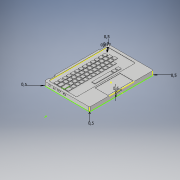
# Autodesk Inventor part: UnderdelDatorchassi
Saved by Autodesk Inventor 2018 (Build 220112000, 112)
## iProperties
Created: 2017-11-21
Part Number: UnderdelDatorchassi
Material: Generic
Document SubType Name: Modeling
Designer: 17riwi
Density: 1 g/cm^3
Appearance: Default
Author: 17riwi
## iProperties of the stored document UnderdelDatorchassi_3DPrint.ipt
Created: 2017-12-14
Part Number: UnderdelDatorchassi_3DPrint
Material: Generic
Document SubType Name: Modeling
Designer: 17riwi
Density: 1 g/cm^3
Appearance: Default
Author: 17riwi
Autodesk Inventor part; units mm, degrees
(part 1 of 2)
ref_plane "YZ Plane" through (0, 0, 0) normal (1, 0, 0) x (0, 1, 0)
ref_plane "XZ Plane" through (0, 0, 0) normal (0, 1, 0) x (-1, 0, 0)
ref_plane "XY Plane" through (0, 0, 0) normal (0, 0, 1) x (1, 0, 0)
sketch "Sketch1" plane through (0, 0, 0) normal (0, 1, 0) x (-1, 0, 0)
  point P0 (0, 0)
sketch "Sketch2" plane through (0, 0, 0) normal (0, 1, 0) x (-1, 0, 0)
  line L0 (-50.8, 147.4) -> (-50.8, -147.4)
  line L1 (-45.8, -152.4) -> (160.1, -152.4)
  line L2 (160.1, 152.4) -> (-45.8, 152.4)
  arc A0 (-45.8, 152.4) -> (-50.8, 147.4) centre (-45.8, 147.4) ccw
  arc A1 (-50.8, -147.4) -> (-45.8, -152.4) centre (-45.8, -147.4) ccw
  arc A2 (160.1, -152.4) -> (165.1, -147.4) centre (160.1, -147.4) ccw
  arc A3 (165.1, 147.4) -> (160.1, 152.4) centre (160.1, 147.4) ccw
  line L3 (160.0443, 130.175) -> (165.1, 130.175)
  line L4 (165.1, 130.175) -> (168.275, 130.175)
  line L5 (168.2193, 130.0929) -> (168.2193, 104.6929)
  line L6 (168.2193, 104.6929) -> (165.1, 104.6929)
  line L7 (160.0443, 104.6929) -> (160.0443, 130.175)
  line L8 (165.1, 130.175) -> (165.1, 147.4)
  line L9 (165.1, 104.6929) -> (160.0443, 104.6929)
  line L10 (161.6875, -106.4446) -> (166.6318, -106.4446)
  line L11 (166.6318, -106.4446) -> (169.8625, -106.4446)
  line L12 (169.8625, -106.4446) -> (169.8625, -131.7625)
  line L13 (169.8625, -131.7625) -> (166.6875, -131.7625)
  line L14 (161.6875, -131.7625) -> (161.6875, -106.4446)
  line L15 (166.6875, -131.7625) -> (161.6875, -131.7625)
  line L16 (171.45, -131.6395) -> (171.45, -131.7625)
  line L17 (165.1, -147.4) -> (165.1, -131.7625)
  line L18 (165.1, -106.4446) -> (165.1, 104.6929)
  line L19 (22.225, -126.9496) -> (22.225, -131.7625)
  line L20 (22.1693, -44.5321) -> (22.1693, -106.4446)
  line L21 (22.225, -131.7625) -> (22.225, -126.9496)
  line L22 (22.1693, -106.4446) -> (22.1693, 104.6929)
  line L23 (22.225, 130.175) -> (22.225, 134.2875)
  line L24 (153.8637, 11.0475) -> (153.8637, 132.4231)
  line L25 (146.8637, 141.2875) -> (29.225, 141.2875)
  line L26 (22.225, 134.2875) -> (22.225, -126.9496)
  arc A4 (153.7963, -127.9188) -> (153.8637, -126.9496) centre (146.8637, -126.9496) ccw
  arc A5 (29.225, 141.2875) -> (22.225, 134.2875) centre (29.225, 134.2875) ccw
  line L27 (-45.8, -60.325) -> (15.875, -60.325)
  line L28 (-19.5021, 60.09) -> (15.875, 60.09)
  line L29 (15.875, 60.09) -> (15.875, -60.325)
  line L30 (-19.05, -60.325) -> (-45.8, -60.325)
  line L31 (-45.8, -60.325) -> (-45.8, 60.09)
  line L32 (-45.8, 60.09) -> (15.875, 60.09)
  line L33 (-14.9625, 60.325) -> (15.875, 60.325)
  line L34 (-9.525, -60.325) -> (15.875, -60.325)
  line L35 (15.875, -60.325) -> (15.875, 60.325)
  line L36 (22.225, -132.5813) -> (22.225, -131.7625)
  line L37 (22.225, -44.45) -> (22.225, -106.3625)
  line L38 (22.225, -131.7625) -> (22.225, -132.5813)
  line L39 (22.225, -106.3625) -> (22.225, 104.775)
  line L40 (22.225, 130.175) -> (22.225, 134.2875)
  line L41 (148.575, -139.5812) -> (29.225, -139.5812)
  line L42 (155.575, -132.5813) -> (155.575, 134.2875)
  line L43 (148.575, 141.2875) -> (29.225, 141.2875)
  line L44 (22.225, 134.2875) -> (22.225, -132.5813)
  arc A6 (148.575, -139.5812) -> (155.575, -132.5813) centre (148.575, -132.5813) ccw
  arc A7 (22.225, -132.5813) -> (29.225, -139.5812) centre (29.225, -132.5813) ccw
  arc A8 (29.225, 141.2875) -> (22.225, 134.2875) centre (29.225, 134.2875) ccw
  arc A9 (155.575, 134.2875) -> (148.575, 141.2875) centre (148.575, 134.2875) ccw
  line L45 (26.9875, 60.325) -> (26.9875, 60.09)
  line L46 (147.2195, 137.8825) -> (31.8081, 137.8825)
  arc A10 (146.8637, -135.8473) -> (153.7963, -127.9188) centre (147.127, -129.0825) ccw
  arc A11 (31.8081, 137.8825) -> (25.0381, 131.1125) centre (31.8081, 131.1125) ccw
  line L47 (26.9875, 60.325) -> (26.9875, 60.09)
  line L48 (146.8637, -135.8473) -> (33.9358, -135.8473)
  arc A12 (25.0381, -126.9496) -> (33.9358, -135.8473) centre (33.9358, -126.9496) ccw
  arc A13 (33.9875, 282.575) -> (31.3881, 282.0745) centre (33.9875, 275.575) ccw
  line L49 (25.0381, 131.1125) -> (25.0381, -126.9496)
  arc A14 (153.8637, 132.4231) -> (147.2195, 137.8825) centre (147.0348, 130.8849) ccw
  line L50 (153.8637, -126.9449) -> (153.8637, 1.7361)
  line L51 (153.9875, 60.09) -> (153.9875, 60.325)
  line L52 (153.8637, 1.7361) -> (153.8637, 11.0475)
  point P0 (0, 0)
  point P1 (22.225, -133.9496)
  point P2 (153.8637, 134.2875)
  point P3 (22.225, -139.5812)
  point P4 (26.9875, 1.7063)
  point P5 (26.9875, 1.7063)
  dimension "d0" = 5
  dimension "d1" = 5
  dimension "d2" = 5
  dimension "d3" = 5
  dimension "d5" = 7
  dimension "d6" = 6.77
  constraints: 106 end point, 31 point on circle, 26 tangent, 23 perpendicular, 19 point on line, 15 centre point, 6 equal radius, 6 vertical, 4 horizontal, 4 parallel, 2 collinear, 1 coincident
  measures "d0" radius of A0
  measures "d1" radius of A1
  measures "d2" radius of A2
  measures "d3" radius of A3
  measures "d5" radius of A6
  measures "d6" radius of A10
extrude "Extrusion1" add sketch "Sketch2" along normal blind 1 contours L31 L32 L28 L29 L27
extrude "Extrusion2" cut sketch "Sketch2" along normal blind 18 contours L31 L32 L28 L29 L27
extrude "Extrusion3" add sketch "Sketch2" along normal blind 19 contours A0 L2 A3 L8 L3 L7 L9 L18 L10 L14 L15 L17 A2 L1 A1 L0
extrude "Extrusion4" add sketch "Sketch2" along normal blind 18 contours L26 L23 A5 L25 L43 A9 L42 A6 L41 A7 L36 L19
extrude "Extrusion5" cut sketch "Sketch2" against normal blind 1 contours L26 L23 A5 L25 L43 A9 L42 A6 L41 A7 L36 L19
extrude "Extrusion6" add sketch "Sketch2" along normal blind 18 contours L31 L32 L28 L29 L27
extrude "Extrusion7" cut sketch "Sketch2" against normal blind 19 contours L26 L23 A5 L25 L43 A9 L42 A6 L41 A7 L36 L19
extrude "Extrusion8" cut sketch "Sketch2" along normal blind 1.5375 contours L26 L23 A5 L25 L43 A9 L42 A6 L41 A7 L36 L19
extrude "Extrusion9" add sketch "Sketch2" against normal blind 1.5375 contours L26 L23 A5 L25 L43 A9 L42 A6 L41 A7 L36 L19
boundary_patch "Boundary Patch1"
boundary_patch "Boundary Patch2"
sketch "Sketch3" plane through (-160.1, 0, 152.4) normal (0, 0, 1) x (1, 0, 0)
  circle A0 centre (19.8438, 12.7) radius 3.9888
  line L0 (36.5125, 12.7) -> (36.5125, 8.7112)
  line L1 (36.5125, 8.7112) -> (46.0375, 8.7112)
  line L2 (46.0375, 8.7112) -> (46.0375, 12.7)
  line L3 (46.0375, 12.7) -> (36.5125, 12.7)
  line L4 (58.7375, 8.7112) -> (55.5625, 12.7)
  line L5 (55.5625, 12.7) -> (55.5625, 14.6944)
  line L6 (58.7375, 8.7112) -> (68.2625, 8.7112)
  line L7 (68.2625, 8.7112) -> (71.4375, 12.7)
  line L8 (71.4375, 12.7) -> (71.4375, 14.6944)
  line L9 (71.4375, 14.6944) -> (55.5625, 14.6944)
  line L10 (84.1375, 14.6944) -> (84.1375, 8.7112)
  line L11 (84.1375, 8.7112) -> (96.8375, 8.7112)
  line L12 (96.8375, 8.7112) -> (96.8375, 14.6944)
  line L13 (96.8375, 14.6944) -> (84.1375, 14.6944)
  point P0 (160.1, 0)
  constraints: 28 end point, 7 perpendicular, 1 centre point, 1 horizontal, 1 vertical
extrude "Extrusion10" cut sketch "Sketch3" against normal blind 5
sketch3d "3D Sketch2"
sketch "Sketch4" plane through (45.8, 0, -152.4) normal (0, 0, -1) x (-1, 0, 0)
  line L0 (0, 19) -> (205.9, 19) projected
  line L1 (192.1104, 15.875) -> (192.1104, 9.525)
  line L2 (192.1104, 9.525) -> (183.6418, 9.525)
  circle A0 centre (186.0563, 12.7) radius 3.9888 projected
  line L3 (183.6418, 15.875) -> (192.1104, 15.875)
  line L4 (183.6418, 15.875) -> (183.6418, 9.525)
  point P0 (45.8, 0)
  constraints: 8 end point, 2 point on circle, 1 parallel, 1 perpendicular, 1 vertical
extrude "Extrusion11" cut sketch "Sketch4" against normal blind 5 contours L1 L2 A0 L3 | A0 L2 L4 L3
sketch "Sketch5" plane through (45.8, 0, -152.4) normal (0, 0, -1) x (-1, 0, 0)
  point P0 (45.8, 0)
sketch "Sketch6" plane through (0, 19, 0) normal (0, 1, 0) x (1, 0, 0)
  point P0 (0, 0)
sketch "Sketch7" plane through (50.8, 0, 147.4) normal (1, 0, 0) x (0, 0, -1)
  line L0 (87.31, 19) -> (207.725, 19) projected
  line L1 (147.5175, 19) -> (147.5175, 13)
  line L2 (294.8, 0) -> (294.8, 19) projected
  line L3 (-5, 0) -> (-5, 19) projected
  point P0 (147.4, 0)
  dimension "d36" = 6
  constraints: 2 end point, 1 midpoint, 1 vertical
  measures "d36" distance of L1.start L1.end
sketch "Sketch8" plane through (0, 18, 0) normal (0, 1, 0) x (1, 0, 0)
  line L0 (-155.575, 132.5813) -> (-155.575, -134.2875) projected
  point P0 (0, 0)
sketch "Sketch9" plane through (0, 18, 0) normal (0, 1, 0) x (1, 0, 0)
  point P0 (0, 0)
sketch "Sketch10" plane through (0, 18, 0) normal (0, 1, 0) x (1, 0, 0)
  point P0 (0, 0)
sketch "Sketch11" plane through (0, 18, 0) normal (0, 1, 0) x (1, 0, 0)
  point P0 (0, 0)
sketch "Sketch12" plane through (0, 18, 0) normal (0, 1, 0) x (1, 0, 0)
  point P0 (0, 0)
sketch "Sketch13" plane through (0, 18, 0) normal (0, 1, 0) x (1, 0, 0)
  line L0 (-136.525, 106.3625) -> (-120.65, 106.3625)
  line L1 (-120.65, 106.3625) -> (-120.65, 90.4875)
  line L2 (-120.65, 90.4875) -> (-136.525, 90.4875)
  line L3 (-136.525, 90.4875) -> (-136.525, 106.3625)
  line L4 (-136.525, 88.9) -> (-120.65, 88.9)
  line L5 (-120.65, 88.9) -> (-120.65, 73.025)
  line L6 (-120.65, 73.025) -> (-136.525, 73.025)
  line L7 (-136.525, 73.025) -> (-136.525, 88.9)
  line L8 (-136.525, 69.85) -> (-120.65, 69.85)
  line L9 (-120.65, 69.85) -> (-120.65, 53.975)
  line L10 (-120.65, 53.975) -> (-136.525, 53.975)
  line L11 (-136.525, 53.975) -> (-136.525, 69.85)
  line L12 (-136.525, 50.8) -> (-120.65, 50.8)
  line L13 (-120.65, 50.8) -> (-120.65, 34.925)
  line L14 (-120.65, 34.925) -> (-136.525, 34.925)
  line L15 (-136.525, 34.925) -> (-136.525, 50.8)
  line L16 (-136.525, 33.3375) -> (-120.65, 33.3375)
  line L17 (-120.65, 33.3375) -> (-120.65, 17.4625)
  line L18 (-120.65, 17.4625) -> (-136.525, 17.4625)
  line L19 (-136.525, 17.4625) -> (-136.525, 33.3375)
  line L20 (-136.525, 15.875) -> (-120.65, 15.875)
  line L21 (-120.65, 15.875) -> (-120.65, 0)
  line L22 (-120.65, 0) -> (-136.525, 0)
  line L23 (-136.525, 0) -> (-136.525, 15.875)
  line L24 (-136.525, -1.5875) -> (-120.65, -1.5875)
  line L25 (-120.65, -1.5875) -> (-120.65, -17.4625)
  line L26 (-120.65, -17.4625) -> (-136.525, -17.4625)
  line L27 (-136.525, -17.4625) -> (-136.525, -1.5875)
  line L28 (-136.525, -19.05) -> (-120.65, -19.05)
  line L29 (-120.65, -19.05) -> (-120.65, -34.925)
  line L30 (-120.65, -34.925) -> (-136.525, -34.925)
  line L31 (-136.525, -34.925) -> (-136.525, -19.05)
  line L32 (-136.525, -38.1) -> (-120.65, -38.1)
  line L33 (-120.65, -38.1) -> (-120.65, -53.975)
  line L34 (-120.65, -53.975) -> (-136.525, -53.975)
  line L35 (-136.525, -53.975) -> (-136.525, -38.1)
  line L36 (-136.525, -55.5625) -> (-120.65, -55.5625)
  line L37 (-120.65, -55.5625) -> (-120.65, -71.4375)
  line L38 (-120.65, -71.4375) -> (-136.525, -71.4375)
  line L39 (-136.525, -71.4375) -> (-136.525, -55.5625)
  line L40 (-136.525, -74.6125) -> (-120.65, -74.6125)
  line L41 (-120.65, -74.6125) -> (-120.65, -90.4875)
  line L42 (-120.65, -90.4875) -> (-136.525, -90.4875)
  line L43 (-136.525, -90.4875) -> (-136.525, -74.6125)
  line L44 (-136.525, -92.075) -> (-120.65, -92.075)
  line L45 (-120.65, -92.075) -> (-120.65, -107.95)
  line L46 (-120.65, -107.95) -> (-136.525, -107.95)
  line L47 (-136.525, -107.95) -> (-136.525, -92.075)
  line L48 (-136.525, -109.5375) -> (-120.65, -109.5375)
  line L49 (-120.65, -109.5375) -> (-120.65, -125.4125)
  line L50 (-120.65, -125.4125) -> (-136.525, -125.4125)
  line L51 (-136.525, -125.4125) -> (-136.525, -109.5375)
  point P0 (0, 0)
  constraints: 104 end point, 26 parallel, 18 point on line, 13 horizontal, 13 perpendicular
extrude "Extrusion12" cut sketch "Sketch13" against normal blind 5
sketch "Sketch14" plane through (0, 18, 0) normal (0, 1, 0) x (1, 0, 0)
  line L0 (-120.65, 50.8) -> (-120.65, 34.925) projected
  line L1 (-117.475, 39.6875) -> (-117.475, 20.6875)
  line L2 (-117.475, 15.6875) -> (-117.475, 1.6875)
  line L3 (-117.475, -3.3125) -> (-117.475, -17.3125)
  line L4 (-117.475, -22.3125) -> (-117.475, -36.3125)
  line L5 (-117.475, -41.3125) -> (-117.475, -55.3125)
  line L6 (-117.475, -60.3125) -> (-117.475, -74.3125)
  line L7 (-117.475, -79.3125) -> (-117.475, -93.223)
  line L8 (-117.475, -93.3125) -> (-117.475, -88.3125)
  line L9 (-117.475, -102.3125) -> (-117.475, -112.223)
  line L10 (-102.475, -102.3125) -> (-102.475, -97.3125)
  line L11 (-102.475, 111.125) -> (-117.475, 111.125)
  line L12 (-117.475, 111.125) -> (-102.475, 111.125)
  line L13 (-117.475, 96.8375) -> (-102.475, 96.8375)
  line L14 (-117.475, 92.075) -> (-102.475, 92.075)
  line L15 (-117.475, 77.7875) -> (-102.475, 77.7875)
  line L16 (-117.475, 73.025) -> (-102.475, 73.025)
  line L17 (-117.475, 58.7375) -> (-102.475, 58.7375)
  line L18 (-117.475, 39.6875) -> (-102.475, 39.6875)
  line L19 (-117.475, 34.6875) -> (-102.475, 34.6875)
  line L20 (-117.475, 20.6875) -> (-102.475, 20.6875)
  line L21 (-117.475, 15.6875) -> (-102.475, 15.6875)
  line L22 (-117.475, 1.6875) -> (-102.475, 1.6875)
  line L23 (-117.475, -3.3125) -> (-102.475, -3.3125)
  line L24 (-117.475, -17.3125) -> (-102.475, -17.3125)
  line L25 (-117.475, -22.3125) -> (-102.475, -22.3125)
  line L26 (-117.475, -36.3125) -> (-102.475, -36.3125)
  line L27 (-117.475, -41.3125) -> (-102.475, -41.3125)
  line L28 (-117.475, -55.3125) -> (-102.475, -55.3125)
  line L29 (-117.475, -60.3125) -> (-102.475, -60.3125)
  line L30 (-117.475, -74.3125) -> (-102.475, -74.3125)
  line L31 (-117.475, -79.3125) -> (-102.475, -79.3125)
  line L32 (-98.475, 110.777) -> (-98.475, 101.777)
  line L33 (-98.475, -107.223) -> (-83.475, -107.223)
  line L34 (-98.475, -107.223) -> (-98.475, -93.3125)
  line L35 (-98.475, -88.223) -> (-98.475, -74.3125)
  line L36 (-98.475, -69.223) -> (-98.475, -55.223)
  line L37 (-98.475, -50.223) -> (-98.475, -36.223)
  line L38 (-98.475, -31.223) -> (-98.475, -17.3125)
  line L39 (-98.475, -12.223) -> (-98.475, 1.777)
  line L40 (-98.475, 6.777) -> (-98.475, 20.777)
  line L41 (-98.475, 25.777) -> (-98.475, 39.777)
  line L42 (-98.475, 44.777) -> (-98.475, 58.777)
  line L43 (-98.475, 63.777) -> (-98.475, 77.777)
  line L44 (-98.475, 77.777) -> (-98.475, 77.7875)
  line L45 (-98.475, 82.777) -> (-98.475, 96.777)
  line L46 (-98.475, 97.777) -> (-98.475, 82.777)
  line L47 (-98.475, 82.777) -> (-98.475, 96.777)
  line L48 (-98.475, 101.777) -> (-98.475, 115.777)
  line L49 (-98.475, 115.777) -> (-83.475, 115.777)
  line L50 (-98.475, 101.777) -> (-83.475, 101.777)
  line L51 (-83.475, 96.777) -> (-98.475, 96.777)
  line L52 (-98.475, 82.777) -> (-83.475, 82.777)
  line L53 (-83.475, 77.777) -> (-98.475, 77.777)
  line L54 (-98.475, 63.777) -> (-83.475, 63.777)
  line L55 (-83.475, 58.777) -> (-98.475, 58.777)
  line L56 (-98.475, 44.777) -> (-83.475, 44.777)
  line L57 (-83.475, 39.777) -> (-98.475, 39.777)
  line L58 (-98.475, 25.777) -> (-83.475, 25.777)
  line L59 (-83.475, 20.777) -> (-98.475, 20.777)
  line L60 (-98.475, 6.777) -> (-83.475, 6.777)
  line L61 (-83.475, 1.777) -> (-98.475, 1.777)
  line L62 (-98.475, -12.223) -> (-83.475, -12.223)
  line L63 (-83.475, -17.223) -> (-98.475, -17.223)
  line L64 (-98.475, -31.223) -> (-83.475, -31.223)
  line L65 (-83.475, -36.223) -> (-98.475, -36.223)
  line L66 (-98.475, -50.223) -> (-83.475, -50.223)
  line L67 (-83.475, -55.223) -> (-98.475, -55.223)
  line L68 (-98.475, -69.223) -> (-83.475, -69.223)
  line L69 (-98.475, -88.223) -> (-83.475, -88.223)
  line L70 (-83.475, -93.223) -> (-98.475, -93.223)
  line L71 (-98.475, -112.223) -> (-83.475, -112.223)
  line L72 (-83.475, -112.223) -> (-83.475, -138.223)
  line L73 (-83.475, -138.223) -> (-98.475, -138.223)
  line L74 (-98.475, -138.223) -> (-98.475, -112.223)
  line L75 (-90.975, 119.936) -> (-83.475, 119.936)
  line L76 (-92.075, 119.936) -> (-83.475, 119.936)
  line L77 (-83.475, 119.936) -> (-83.475, 132.936)
  line L78 (-83.475, 132.936) -> (-117.475, 132.936)
  line L79 (-117.475, 132.936) -> (-117.475, 115.936)
  line L80 (-117.475, 115.936) -> (-117.475, 132.936)
  line L81 (-83.475, -107.223) -> (-98.475, -107.223)
  line L82 (-98.475, -107.223) -> (-98.475, -93.223)
  line L83 (-98.475, -93.223) -> (-83.475, -93.223)
  line L84 (-83.475, -93.223) -> (-83.475, -107.223)
  line L85 (-83.475, -88.223) -> (-98.475, -88.223)
  line L86 (-98.475, -88.223) -> (-98.475, -74.223)
  line L87 (-98.475, -74.223) -> (-83.475, -74.223)
  line L88 (-83.475, -74.223) -> (-83.475, -88.223)
  line L89 (-83.475, -69.223) -> (-98.475, -69.223)
  line L90 (-98.475, -69.223) -> (-98.475, -55.223)
  line L91 (-98.475, -55.223) -> (-83.475, -55.223)
  line L92 (-83.475, -55.223) -> (-83.475, -69.223)
  line L93 (-83.475, -50.223) -> (-98.475, -50.223)
  line L94 (-98.475, -50.223) -> (-98.475, -36.223)
  line L95 (-98.475, -36.223) -> (-83.475, -36.223)
  line L96 (-83.475, -36.223) -> (-83.475, -50.223)
  line L97 (-83.475, -31.223) -> (-98.475, -31.223)
  line L98 (-98.475, -31.223) -> (-98.475, -17.223)
  line L99 (-98.475, -17.223) -> (-83.475, -17.223)
  line L100 (-83.475, -17.223) -> (-83.475, -31.223)
  line L101 (-83.475, -12.223) -> (-98.475, -12.223)
  line L102 (-98.475, -12.223) -> (-98.475, 1.777)
  line L103 (-98.475, 1.777) -> (-83.475, 1.777)
  line L104 (-83.475, 1.777) -> (-83.475, -12.223)
  line L105 (-83.475, 6.777) -> (-98.475, 6.777)
  line L106 (-98.475, 6.777) -> (-98.475, 20.6875)
  line L107 (-98.475, 20.777) -> (-83.475, 20.777)
  line L108 (-83.475, 20.777) -> (-83.475, 20.6875)
  line L109 (-83.475, 25.777) -> (-98.475, 25.777)
  line L110 (-98.475, 25.777) -> (-98.475, 39.777)
  line L111 (-98.475, 39.777) -> (-83.475, 39.777)
  line L112 (-83.475, 39.777) -> (-83.475, 25.777)
  line L113 (-83.475, 44.777) -> (-98.475, 44.777)
  line L114 (-98.475, 44.777) -> (-98.475, 58.777)
  line L115 (-98.475, 58.777) -> (-83.475, 58.777)
  line L116 (-83.475, 58.777) -> (-83.475, 44.777)
  line L117 (-83.475, 63.777) -> (-98.475, 63.777)
  line L118 (-98.475, 63.777) -> (-98.475, 77.777)
  line L119 (-98.475, 77.777) -> (-83.475, 77.777)
  line L120 (-83.475, 77.777) -> (-83.475, 63.777)
  line L121 (-83.475, 82.777) -> (-98.475, 82.777)
  line L122 (-98.475, 82.777) -> (-98.475, 96.777)
  line L123 (-98.475, 96.777) -> (-83.475, 96.777)
  line L124 (-83.475, 96.777) -> (-83.475, 82.777)
  line L125 (-83.475, 101.777) -> (-98.475, 101.777)
  line L126 (-98.475, 101.777) -> (-98.475, 115.777)
  line L127 (-98.475, 115.777) -> (-83.475, 115.777)
  line L128 (-83.475, 115.777) -> (-83.475, 101.777)
  line L129 (-83.475, -112.223) -> (-98.475, -112.223)
  line L130 (-98.475, -112.223) -> (-98.475, -138.223)
  line L131 (-98.475, -138.223) -> (-83.475, -138.223)
  line L132 (-83.475, -138.223) -> (-83.475, -112.223)
  line L133 (-102.475, 111.125) -> (-117.475, 111.125)
  line L134 (-117.475, 111.125) -> (-117.475, 96.8375)
  line L135 (-117.475, 96.8375) -> (-102.475, 96.8375)
  line L136 (-102.475, 96.8375) -> (-102.475, 111.125)
  line L137 (-102.475, 92.075) -> (-117.475, 92.075)
  line L138 (-117.475, 92.075) -> (-117.475, 77.7875)
  line L139 (-117.475, 77.7875) -> (-102.475, 77.7875)
  line L140 (-102.475, 77.7875) -> (-102.475, 92.075)
  line L141 (-102.475, 73.025) -> (-117.475, 73.025)
  line L142 (-117.475, 73.025) -> (-117.475, 58.7375)
  line L143 (-117.475, 58.7375) -> (-102.475, 58.7375)
  line L144 (-102.475, 58.7375) -> (-102.475, 73.025)
  line L145 (-102.475, 53.975) -> (-117.475, 53.975)
  line L146 (-117.475, 53.975) -> (-117.475, 39.6875)
  line L147 (-117.475, 39.6875) -> (-102.475, 39.6875)
  line L148 (-102.475, 39.6875) -> (-102.475, 53.975)
  line L149 (-102.475, 34.6875) -> (-117.475, 34.6875)
  line L150 (-117.475, 34.6875) -> (-117.475, 20.6875)
  line L151 (-117.475, 20.6875) -> (-102.475, 20.6875)
  line L152 (-102.475, 20.6875) -> (-102.475, 34.6875)
  line L153 (-102.475, 15.6875) -> (-117.475, 15.6875)
  line L154 (-117.475, 15.6875) -> (-117.475, 1.6875)
  line L155 (-117.475, 1.6875) -> (-102.475, 1.6875)
  line L156 (-102.475, 1.6875) -> (-102.475, 15.6875)
  line L157 (-102.475, -3.3125) -> (-117.475, -3.3125)
  line L158 (-117.475, -3.3125) -> (-117.475, -17.3125)
  line L159 (-117.475, -17.3125) -> (-102.475, -17.3125)
  line L160 (-102.475, -17.3125) -> (-102.475, -17.223)
  line L161 (-102.475, -22.3125) -> (-117.475, -22.3125)
  line L162 (-117.475, -22.3125) -> (-117.475, -36.3125)
  line L163 (-117.475, -36.3125) -> (-102.475, -36.3125)
  line L164 (-102.475, -36.3125) -> (-102.475, -22.3125)
  line L165 (-102.475, -41.3125) -> (-117.475, -41.3125)
  line L166 (-117.475, -41.3125) -> (-117.475, -55.3125)
  line L167 (-117.475, -55.3125) -> (-102.475, -55.3125)
  line L168 (-102.475, -55.3125) -> (-102.475, -55.223)
  line L169 (-102.475, -60.3125) -> (-117.475, -60.3125)
  line L170 (-117.475, -60.3125) -> (-117.475, -74.3125)
  line L171 (-117.475, -74.3125) -> (-102.475, -74.3125)
  line L172 (-102.475, -74.3125) -> (-102.475, -74.223)
  line L173 (-102.475, -79.3125) -> (-117.475, -79.3125)
  line L174 (-117.475, -79.3125) -> (-117.475, -93.3125)
  line L175 (-102.475, -93.3125) -> (-102.475, -79.3125)
  line L176 (-83.475, -107.223) -> (-83.475, -93.223)
  line L177 (-83.475, 25.777) -> (-83.475, 39.777)
  line L178 (-98.475, 20.6875) -> (-98.475, 20.777)
  line L179 (-98.475, 58.777) -> (-98.475, 44.777)
  line L180 (-98.475, 96.777) -> (-98.475, 97.777)
  line L181 (-98.475, 1.777) -> (-98.475, -12.223)
  line L182 (-98.475, -17.3125) -> (-98.475, -17.223)
  line L183 (-98.475, -36.223) -> (-98.475, -50.223)
  line L184 (-98.475, -55.223) -> (-98.475, -69.223)
  line L185 (-98.475, -74.3125) -> (-98.475, -74.223)
  line L186 (-98.475, -88.3125) -> (-98.475, -88.223)
  line L187 (-98.475, -93.3125) -> (-98.475, -93.223)
  line L188 (-98.475, -93.223) -> (-98.475, -107.223)
  line L189 (-83.475, -88.223) -> (-83.475, -74.223)
  line L190 (-83.475, -69.223) -> (-83.475, -55.223)
  line L191 (-83.475, -50.223) -> (-83.475, -36.223)
  line L192 (-83.475, -31.223) -> (-83.475, -17.223)
  line L193 (-83.475, -12.223) -> (-83.475, 1.777)
  line L194 (-83.475, 6.777) -> (-83.475, 20.777)
  line L195 (-83.475, 20.6875) -> (-83.475, 6.777)
  line L196 (-83.475, 44.777) -> (-83.475, 58.777)
  line L197 (-83.475, 63.777) -> (-83.475, 77.777)
  line L198 (-83.475, 82.777) -> (-83.475, 96.777)
  line L199 (-83.475, 101.777) -> (-83.475, 115.777)
  line L200 (-102.475, 96.8375) -> (-102.475, 111.125)
  line L201 (-102.475, 96.777) -> (-102.475, 96.8375)
  line L202 (-102.475, 77.7875) -> (-102.475, 92.075)
  line L203 (-102.475, 77.777) -> (-102.475, 77.7875)
  line L204 (-102.475, 58.7375) -> (-102.475, 73.025)
  line L205 (-102.475, 39.6875) -> (-102.475, 53.975)
  line L206 (-102.475, 20.6875) -> (-102.475, 34.6875)
  line L207 (-102.475, 1.6875) -> (-102.475, 15.6875)
  line L208 (-102.475, -17.223) -> (-102.475, -3.3125)
  line L209 (-102.475, -17.3125) -> (-102.475, -3.3125)
  line L210 (-102.475, -36.3125) -> (-102.475, -22.3125)
  line L211 (-102.475, -55.223) -> (-102.475, -41.3125)
  line L212 (-102.475, -74.223) -> (-102.475, -60.3125)
  line L213 (-102.475, -102.3125) -> (-102.475, -97.3125)
  line L214 (-102.475, -97.3125) -> (-117.475, -97.3125)
  line L215 (-102.475, -79.3125) -> (-102.475, -93.3125)
  line L216 (-102.475, -93.3125) -> (-117.475, -93.3125)
  line L217 (-102.475, -97.3125) -> (-102.475, -111.3125)
  line L218 (-102.475, -111.3125) -> (-117.475, -112.223)
  line L219 (-117.475, -112.223) -> (-102.475, -112.223)
  line L220 (-102.475, -112.223) -> (-102.475, -97.3125)
  line L221 (-102.475, -97.3125) -> (-117.475, -97.3125)
  line L222 (-117.475, -97.3125) -> (-117.475, -112.223)
  line L223 (-102.475, -93.3125) -> (-102.475, -79.3125)
  line L224 (-117.475, -93.223) -> (-117.475, -93.3125)
  line L225 (-117.475, -97.3125) -> (-117.475, -102.3125)
  line L226 (-102.475, -111.3125) -> (-102.475, -102.3125)
  line L227 (-102.475, -138.223) -> (-102.475, -117.223)
  line L228 (-102.475, -117.223) -> (-117.475, -117.223)
  line L229 (-117.475, -117.223) -> (-117.475, -138.223)
  line L230 (-117.475, -138.223) -> (-102.475, -138.223)
  line L231 (-29.225, -141.2875) -> (-148.575, -141.2875) projected
  line L232 (-80.0875, 86.2375) -> (-80.0875, 77.2375)
  line L233 (-80.0875, -93.7625) -> (-80.0875, -79.7625)
  line L234 (-80.0875, -74.7625) -> (-80.0875, -60.7625)
  line L235 (-80.0875, -55.7625) -> (-80.0875, -41.852)
  line L236 (-80.0875, -36.7625) -> (-80.0875, -22.7625)
  line L237 (-80.0875, -17.7625) -> (-80.0875, -3.7625)
  line L238 (-80.0875, 1.2375) -> (-80.0875, 15.2375)
  line L239 (-80.0875, 20.2375) -> (-80.0875, 34.2375)
  line L240 (-80.0875, 39.2375) -> (-80.0875, 53.2375)
  line L241 (-80.0875, 53.2375) -> (-80.0875, 53.248)
  line L242 (-80.0875, 58.2375) -> (-80.0875, 72.2375)
  line L243 (-80.0875, 73.2375) -> (-80.0875, 58.2375)
  line L244 (-80.0875, 58.2375) -> (-80.0875, 72.2375)
  line L245 (-80.0875, 77.2375) -> (-80.0875, 91.2375)
  line L246 (-80.0875, 91.2375) -> (-65.0875, 91.2375)
  line L247 (-80.0875, 77.2375) -> (-65.0875, 77.2375)
  line L248 (-65.0875, 72.2375) -> (-80.0875, 72.2375)
  line L249 (-80.0875, 58.2375) -> (-65.0875, 58.2375)
  line L250 (-65.0875, 53.2375) -> (-80.0875, 53.2375)
  line L251 (-80.0875, 39.2375) -> (-65.0875, 39.2375)
  line L252 (-65.0875, 34.2375) -> (-80.0875, 34.2375)
  line L253 (-80.0875, 20.2375) -> (-65.0875, 20.2375)
  line L254 (-65.0875, 15.2375) -> (-80.0875, 15.2375)
  line L255 (-80.0875, 1.2375) -> (-65.0875, 1.2375)
  line L256 (-65.0875, -3.7625) -> (-80.0875, -3.7625)
  line L257 (-80.0875, -17.7625) -> (-65.0875, -17.7625)
  line L258 (-65.0875, -22.7625) -> (-80.0875, -22.7625)
  line L259 (-80.0875, -36.7625) -> (-65.0875, -36.7625)
  line L260 (-65.0875, -41.7625) -> (-80.0875, -41.7625)
  line L261 (-80.0875, -55.7625) -> (-65.0875, -55.7625)
  line L262 (-65.0875, -60.7625) -> (-80.0875, -60.7625)
  line L263 (-80.0875, -74.7625) -> (-65.0875, -74.7625)
  line L264 (-65.0875, -79.7625) -> (-80.0875, -79.7625)
  line L265 (-80.0875, -93.7625) -> (-65.0875, -93.7625)
  line L266 (-65.0875, -93.7625) -> (-80.0875, -93.7625)
  line L267 (-80.0875, -93.7625) -> (-80.0875, -79.7625)
  line L268 (-80.0875, -79.7625) -> (-65.0875, -79.7625)
  line L269 (-65.0875, -79.7625) -> (-65.0875, -93.7625)
  line L270 (-65.0875, -74.7625) -> (-80.0875, -74.7625)
  line L271 (-80.0875, -74.7625) -> (-80.0875, -60.7625)
  line L272 (-80.0875, -60.7625) -> (-65.0875, -60.7625)
  line L273 (-65.0875, -60.7625) -> (-65.0875, -74.7625)
  line L274 (-65.0875, -55.7625) -> (-80.0875, -55.7625)
  line L275 (-80.0875, -55.7625) -> (-80.0875, -41.7625)
  line L276 (-80.0875, -41.7625) -> (-65.0875, -41.7625)
  line L277 (-65.0875, -41.7625) -> (-65.0875, -55.7625)
  line L278 (-65.0875, -36.7625) -> (-80.0875, -36.7625)
  line L279 (-80.0875, -36.7625) -> (-80.0875, -22.7625)
  line L280 (-80.0875, -22.7625) -> (-65.0875, -22.7625)
  line L281 (-65.0875, -22.7625) -> (-65.0875, -36.7625)
  line L282 (-65.0875, -17.7625) -> (-80.0875, -17.7625)
  line L283 (-80.0875, -17.7625) -> (-80.0875, -3.852)
  line L284 (-80.0875, -3.7625) -> (-65.0875, -3.7625)
  line L285 (-65.0875, -3.7625) -> (-65.0875, -3.852)
  line L286 (-65.0875, 1.2375) -> (-80.0875, 1.2375)
  line L287 (-80.0875, 1.2375) -> (-80.0875, 15.2375)
  line L288 (-80.0875, 15.2375) -> (-65.0875, 15.2375)
  line L289 (-65.0875, 15.2375) -> (-65.0875, 1.2375)
  line L290 (-65.0875, 20.2375) -> (-80.0875, 20.2375)
  line L291 (-80.0875, 20.2375) -> (-80.0875, 34.2375)
  line L292 (-80.0875, 34.2375) -> (-65.0875, 34.2375)
  line L293 (-65.0875, 34.2375) -> (-65.0875, 20.2375)
  line L294 (-65.0875, 39.2375) -> (-80.0875, 39.2375)
  line L295 (-80.0875, 39.2375) -> (-80.0875, 53.2375)
  line L296 (-80.0875, 53.2375) -> (-65.0875, 53.2375)
  line L297 (-65.0875, 53.2375) -> (-65.0875, 39.2375)
  line L298 (-65.0875, 58.2375) -> (-80.0875, 58.2375)
  line L299 (-80.0875, 58.2375) -> (-80.0875, 72.2375)
  line L300 (-80.0875, 72.2375) -> (-65.0875, 72.2375)
  line L301 (-65.0875, 72.2375) -> (-65.0875, 58.2375)
  line L302 (-65.0875, 77.2375) -> (-80.0875, 77.2375)
  line L303 (-80.0875, 77.2375) -> (-80.0875, 91.2375)
  line L304 (-80.0875, 91.2375) -> (-65.0875, 91.2375)
  line L305 (-65.0875, 91.2375) -> (-65.0875, 77.2375)
  line L306 (-65.0875, 1.2375) -> (-65.0875, 15.2375)
  line L307 (-80.0875, -3.852) -> (-80.0875, -3.7625)
  line L308 (-80.0875, 34.2375) -> (-80.0875, 20.2375)
  line L309 (-80.0875, 72.2375) -> (-80.0875, 73.2375)
  line L310 (-80.0875, -22.7625) -> (-80.0875, -36.7625)
  line L311 (-80.0875, -41.852) -> (-80.0875, -41.7625)
  line L312 (-80.0875, -60.7625) -> (-80.0875, -74.7625)
  line L313 (-80.0875, -79.7625) -> (-80.0875, -93.7625)
  line L314 (-65.0875, -93.7625) -> (-65.0875, -79.7625)
  line L315 (-65.0875, -74.7625) -> (-65.0875, -60.7625)
  line L316 (-65.0875, -55.7625) -> (-65.0875, -41.7625)
  line L317 (-65.0875, -36.7625) -> (-65.0875, -22.7625)
  line L318 (-65.0875, -17.7625) -> (-65.0875, -3.7625)
  line L319 (-65.0875, -3.852) -> (-65.0875, -17.7625)
  line L320 (-65.0875, 20.2375) -> (-65.0875, 34.2375)
  line L321 (-65.0875, 39.2375) -> (-65.0875, 53.2375)
  line L322 (-65.0875, 58.2375) -> (-65.0875, 72.2375)
  line L323 (-65.0875, 77.2375) -> (-65.0875, 91.2375)
  line L324 (-80.0875, 86.2375) -> (-80.0875, 77.2375)
  line L325 (-80.0875, -93.7625) -> (-80.0875, -79.7625)
  line L326 (-80.0875, -74.7625) -> (-80.0875, -60.7625)
  line L327 (-80.0875, -55.7625) -> (-80.0875, -41.852)
  line L328 (-80.0875, -36.7625) -> (-80.0875, -22.7625)
  line L329 (-80.0875, -17.7625) -> (-80.0875, -3.7625)
  line L330 (-80.0875, 1.2375) -> (-80.0875, 15.2375)
  line L331 (-80.0875, 20.2375) -> (-80.0875, 34.2375)
  line L332 (-80.0875, 39.2375) -> (-80.0875, 53.2375)
  line L333 (-80.0875, 53.2375) -> (-80.0875, 53.248)
  line L334 (-80.0875, 58.2375) -> (-80.0875, 72.2375)
  line L335 (-80.0875, 73.2375) -> (-80.0875, 58.2375)
  line L336 (-80.0875, 58.2375) -> (-80.0875, 72.2375)
  line L337 (-80.0875, 77.2375) -> (-80.0875, 91.2375)
  line L338 (-80.0875, 91.2375) -> (-65.0875, 91.2375)
  line L339 (-80.0875, 77.2375) -> (-65.0875, 77.2375)
  line L340 (-65.0875, 72.2375) -> (-80.0875, 72.2375)
  line L341 (-80.0875, 58.2375) -> (-65.0875, 58.2375)
  line L342 (-65.0875, 53.2375) -> (-80.0875, 53.2375)
  line L343 (-80.0875, 39.2375) -> (-65.0875, 39.2375)
  line L344 (-65.0875, 34.2375) -> (-80.0875, 34.2375)
  line L345 (-80.0875, 20.2375) -> (-65.0875, 20.2375)
  line L346 (-65.0875, 15.2375) -> (-80.0875, 15.2375)
  line L347 (-80.0875, 1.2375) -> (-65.0875, 1.2375)
  line L348 (-65.0875, -3.7625) -> (-80.0875, -3.7625)
  line L349 (-80.0875, -17.7625) -> (-65.0875, -17.7625)
  line L350 (-65.0875, -22.7625) -> (-80.0875, -22.7625)
  line L351 (-80.0875, -36.7625) -> (-65.0875, -36.7625)
  line L352 (-65.0875, -41.7625) -> (-80.0875, -41.7625)
  line L353 (-80.0875, -55.7625) -> (-65.0875, -55.7625)
  line L354 (-65.0875, -60.7625) -> (-80.0875, -60.7625)
  line L355 (-80.0875, -74.7625) -> (-65.0875, -74.7625)
  line L356 (-65.0875, -79.7625) -> (-80.0875, -79.7625)
  line L357 (-80.0875, -93.7625) -> (-65.0875, -93.7625)
  line L358 (-65.0875, -93.7625) -> (-80.0875, -93.7625)
  line L359 (-80.0875, -93.7625) -> (-80.0875, -79.7625)
  line L360 (-80.0875, -79.7625) -> (-65.0875, -79.7625)
  line L361 (-65.0875, -79.7625) -> (-65.0875, -93.7625)
  line L362 (-65.0875, -74.7625) -> (-80.0875, -74.7625)
  line L363 (-80.0875, -74.7625) -> (-80.0875, -60.7625)
  line L364 (-80.0875, -60.7625) -> (-65.0875, -60.7625)
  line L365 (-65.0875, -60.7625) -> (-65.0875, -74.7625)
  line L366 (-65.0875, -55.7625) -> (-80.0875, -55.7625)
  line L367 (-80.0875, -55.7625) -> (-80.0875, -41.7625)
  line L368 (-80.0875, -41.7625) -> (-65.0875, -41.7625)
  line L369 (-65.0875, -41.7625) -> (-65.0875, -55.7625)
  line L370 (-65.0875, -36.7625) -> (-80.0875, -36.7625)
  line L371 (-80.0875, -36.7625) -> (-80.0875, -22.7625)
  line L372 (-80.0875, -22.7625) -> (-65.0875, -22.7625)
  line L373 (-65.0875, -22.7625) -> (-65.0875, -36.7625)
  line L374 (-65.0875, -17.7625) -> (-80.0875, -17.7625)
  line L375 (-80.0875, -17.7625) -> (-80.0875, -3.852)
  line L376 (-80.0875, -3.7625) -> (-65.0875, -3.7625)
  line L377 (-65.0875, -3.7625) -> (-65.0875, -3.852)
  line L378 (-65.0875, 1.2375) -> (-80.0875, 1.2375)
  line L379 (-80.0875, 1.2375) -> (-80.0875, 15.2375)
  line L380 (-80.0875, 15.2375) -> (-65.0875, 15.2375)
  line L381 (-65.0875, 15.2375) -> (-65.0875, 1.2375)
  line L382 (-65.0875, 20.2375) -> (-80.0875, 20.2375)
  line L383 (-80.0875, 20.2375) -> (-80.0875, 34.2375)
  line L384 (-80.0875, 34.2375) -> (-65.0875, 34.2375)
  line L385 (-65.0875, 34.2375) -> (-65.0875, 20.2375)
  line L386 (-65.0875, 39.2375) -> (-80.0875, 39.2375)
  line L387 (-80.0875, 39.2375) -> (-80.0875, 53.2375)
  line L388 (-80.0875, 53.2375) -> (-65.0875, 53.2375)
  line L389 (-65.0875, 53.2375) -> (-65.0875, 39.2375)
  line L390 (-65.0875, 58.2375) -> (-80.0875, 58.2375)
  line L391 (-80.0875, 58.2375) -> (-80.0875, 72.2375)
  line L392 (-80.0875, 72.2375) -> (-65.0875, 72.2375)
  line L393 (-65.0875, 72.2375) -> (-65.0875, 58.2375)
  line L394 (-65.0875, 77.2375) -> (-80.0875, 77.2375)
  line L395 (-80.0875, 77.2375) -> (-80.0875, 91.2375)
  line L396 (-80.0875, 91.2375) -> (-65.0875, 91.2375)
  line L397 (-65.0875, 91.2375) -> (-65.0875, 77.2375)
  line L398 (-65.0875, 1.2375) -> (-65.0875, 15.2375)
  line L399 (-80.0875, -3.852) -> (-80.0875, -3.7625)
  line L400 (-80.0875, 34.2375) -> (-80.0875, 20.2375)
  line L401 (-80.0875, 72.2375) -> (-80.0875, 73.2375)
  line L402 (-80.0875, -22.7625) -> (-80.0875, -36.7625)
  line L403 (-80.0875, -41.852) -> (-80.0875, -41.7625)
  line L404 (-80.0875, -60.7625) -> (-80.0875, -74.7625)
  line L405 (-80.0875, -79.7625) -> (-80.0875, -93.7625)
  line L406 (-65.0875, -93.7625) -> (-65.0875, -79.7625)
  line L407 (-65.0875, -74.7625) -> (-65.0875, -60.7625)
  line L408 (-65.0875, -55.7625) -> (-65.0875, -41.7625)
  line L409 (-65.0875, -36.7625) -> (-65.0875, -22.7625)
  line L410 (-65.0875, -17.7625) -> (-65.0875, -3.7625)
  line L411 (-65.0875, -3.852) -> (-65.0875, -17.7625)
  line L412 (-65.0875, 20.2375) -> (-65.0875, 34.2375)
  line L413 (-65.0875, 39.2375) -> (-65.0875, 53.2375)
  line L414 (-65.0875, 58.2375) -> (-65.0875, 72.2375)
  line L415 (-65.0875, 77.2375) -> (-65.0875, 91.2375)
  line L416 (-98.475, 110.777) -> (-98.475, 101.777)
  line L417 (-98.475, -107.223) -> (-83.475, -107.223)
  line L418 (-98.475, -107.223) -> (-98.475, -93.3125)
  line L419 (-98.475, -88.223) -> (-98.475, -74.3125)
  line L420 (-98.475, -69.223) -> (-98.475, -55.223)
  line L421 (-98.475, -50.223) -> (-98.475, -36.223)
  line L422 (-98.475, -31.223) -> (-98.475, -17.3125)
  line L423 (-98.475, -12.223) -> (-98.475, 1.777)
  line L424 (-98.475, 6.777) -> (-98.475, 20.777)
  line L425 (-98.475, 25.777) -> (-98.475, 39.777)
  line L426 (-98.475, 44.777) -> (-98.475, 58.777)
  line L427 (-98.475, 63.777) -> (-98.475, 77.777)
  line L428 (-98.475, 77.777) -> (-98.475, 77.7875)
  line L429 (-98.475, 82.777) -> (-98.475, 96.777)
  line L430 (-98.475, 97.777) -> (-98.475, 82.777)
  line L431 (-98.475, 82.777) -> (-98.475, 96.777)
  line L432 (-98.475, 101.777) -> (-98.475, 115.777)
  line L433 (-98.475, 115.777) -> (-83.475, 115.777)
  line L434 (-98.475, 101.777) -> (-83.475, 101.777)
  line L435 (-83.475, 96.777) -> (-98.475, 96.777)
  line L436 (-98.475, 82.777) -> (-83.475, 82.777)
  line L437 (-83.475, 77.777) -> (-98.475, 77.777)
  line L438 (-98.475, 63.777) -> (-83.475, 63.777)
  line L439 (-83.475, 58.777) -> (-98.475, 58.777)
  line L440 (-98.475, 44.777) -> (-83.475, 44.777)
  line L441 (-83.475, 39.777) -> (-98.475, 39.777)
  line L442 (-98.475, 25.777) -> (-83.475, 25.777)
  line L443 (-83.475, 20.777) -> (-98.475, 20.777)
  line L444 (-98.475, 6.777) -> (-83.475, 6.777)
  line L445 (-83.475, 1.777) -> (-98.475, 1.777)
  line L446 (-98.475, -12.223) -> (-83.475, -12.223)
  line L447 (-83.475, -17.223) -> (-98.475, -17.223)
  line L448 (-98.475, -31.223) -> (-83.475, -31.223)
  line L449 (-83.475, -36.223) -> (-98.475, -36.223)
  line L450 (-98.475, -50.223) -> (-83.475, -50.223)
  line L451 (-83.475, -55.223) -> (-98.475, -55.223)
  line L452 (-98.475, -69.223) -> (-83.475, -69.223)
  line L453 (-98.475, -88.223) -> (-83.475, -88.223)
  line L454 (-83.475, -93.223) -> (-98.475, -93.223)
  line L455 (-83.475, -107.223) -> (-98.475, -107.223)
  line L456 (-98.475, -107.223) -> (-98.475, -93.223)
  line L457 (-98.475, -93.223) -> (-83.475, -93.223)
  line L458 (-83.475, -93.223) -> (-83.475, -107.223)
  line L459 (-83.475, -88.223) -> (-98.475, -88.223)
  line L460 (-98.475, -88.223) -> (-98.475, -74.223)
  line L461 (-98.475, -74.223) -> (-83.475, -74.223)
  line L462 (-83.475, -74.223) -> (-83.475, -88.223)
  line L463 (-83.475, -69.223) -> (-98.475, -69.223)
  line L464 (-98.475, -69.223) -> (-98.475, -55.223)
  line L465 (-98.475, -55.223) -> (-83.475, -55.223)
  line L466 (-83.475, -55.223) -> (-83.475, -69.223)
  line L467 (-83.475, -50.223) -> (-98.475, -50.223)
  line L468 (-98.475, -50.223) -> (-98.475, -36.223)
  line L469 (-98.475, -36.223) -> (-83.475, -36.223)
  line L470 (-83.475, -36.223) -> (-83.475, -50.223)
  line L471 (-83.475, -31.223) -> (-98.475, -31.223)
  line L472 (-98.475, -31.223) -> (-98.475, -17.223)
  line L473 (-98.475, -17.223) -> (-83.475, -17.223)
  line L474 (-83.475, -17.223) -> (-83.475, -31.223)
  line L475 (-83.475, -12.223) -> (-98.475, -12.223)
  line L476 (-98.475, -12.223) -> (-98.475, 1.777)
  line L477 (-98.475, 1.777) -> (-83.475, 1.777)
  line L478 (-83.475, 1.777) -> (-83.475, -12.223)
  line L479 (-83.475, 6.777) -> (-98.475, 6.777)
  line L480 (-98.475, 6.777) -> (-98.475, 20.6875)
  line L481 (-98.475, 20.777) -> (-83.475, 20.777)
  line L482 (-83.475, 20.777) -> (-83.475, 20.6875)
  line L483 (-83.475, 25.777) -> (-98.475, 25.777)
  line L484 (-98.475, 25.777) -> (-98.475, 39.777)
  line L485 (-98.475, 39.777) -> (-83.475, 39.777)
  line L486 (-83.475, 39.777) -> (-83.475, 25.777)
  line L487 (-83.475, 44.777) -> (-98.475, 44.777)
  line L488 (-98.475, 44.777) -> (-98.475, 58.777)
  line L489 (-98.475, 58.777) -> (-83.475, 58.777)
  line L490 (-83.475, 58.777) -> (-83.475, 44.777)
  line L491 (-83.475, 63.777) -> (-98.475, 63.777)
  line L492 (-98.475, 63.777) -> (-98.475, 77.777)
  line L493 (-98.475, 77.777) -> (-83.475, 77.777)
  line L494 (-83.475, 77.777) -> (-83.475, 63.777)
  line L495 (-83.475, 82.777) -> (-98.475, 82.777)
  line L496 (-98.475, 82.777) -> (-98.475, 96.777)
  line L497 (-98.475, 96.777) -> (-83.475, 96.777)
  line L498 (-83.475, 96.777) -> (-83.475, 82.777)
  line L499 (-83.475, 101.777) -> (-98.475, 101.777)
  line L500 (-98.475, 101.777) -> (-98.475, 115.777)
  line L501 (-98.475, 115.777) -> (-83.475, 115.777)
  line L502 (-83.475, 115.777) -> (-83.475, 101.777)
  line L503 (-83.475, -107.223) -> (-83.475, -93.223)
  line L504 (-83.475, 25.777) -> (-83.475, 39.777)
  line L505 (-98.475, 20.6875) -> (-98.475, 20.777)
  line L506 (-98.475, 58.777) -> (-98.475, 44.777)
  line L507 (-98.475, 96.777) -> (-98.475, 97.777)
  line L508 (-98.475, 1.777) -> (-98.475, -12.223)
  line L509 (-98.475, -17.3125) -> (-98.475, -17.223)
  line L510 (-98.475, -36.223) -> (-98.475, -50.223)
  line L511 (-98.475, -55.223) -> (-98.475, -69.223)
  line L512 (-98.475, -74.3125) -> (-98.475, -74.223)
  line L513 (-98.475, -88.3125) -> (-98.475, -88.223)
  line L514 (-98.475, -93.3125) -> (-98.475, -93.223)
  line L515 (-98.475, -93.223) -> (-98.475, -107.223)
  line L516 (-83.475, -88.223) -> (-83.475, -74.223)
  line L517 (-83.475, -69.223) -> (-83.475, -55.223)
  line L518 (-83.475, -50.223) -> (-83.475, -36.223)
  line L519 (-83.475, -31.223) -> (-83.475, -17.223)
  line L520 (-83.475, -12.223) -> (-83.475, 1.777)
  line L521 (-83.475, 6.777) -> (-83.475, 20.777)
  line L522 (-83.475, 20.6875) -> (-83.475, 6.777)
  line L523 (-83.475, 44.777) -> (-83.475, 58.777)
  line L524 (-83.475, 63.777) -> (-83.475, 77.777)
  line L525 (-83.475, 82.777) -> (-83.475, 96.777)
  line L526 (-83.475, 101.777) -> (-83.475, 115.777)
  point P0 (0, 0)
  dimension "d82" = 5
  dimension "d83" = 19
  dimension "d84" = 5
  dimension "d85" = 14
  dimension "d86" = 5
  dimension "d87" = 14
  dimension "d88" = 5
  dimension "d89" = 14
  dimension "d90" = 5
  dimension "d91" = 14
  dimension "d92" = 5
  dimension "d93" = 14
  dimension "d94" = 5
  dimension "d95" = 14
  dimension "d97" = 14
  dimension "d105" = 5
  dimension "d106" = 14
  dimension "d107" = 5
  dimension "d108" = 14
  dimension "d109" = 5
  dimension "d110" = 14
  dimension "d111" = 5
  dimension "d112" = 14
  dimension "d114" = 14
  dimension "d115" = 5
  dimension "d116" = 14
  dimension "d117" = 5
  dimension "d119" = 5
  dimension "d120" = 14
  dimension "d121" = 5
  dimension "d122" = 14
  dimension "d123" = 5
  dimension "d125" = 14
  dimension "d126" = 5
  dimension "d127" = 14
  dimension "d130" = 26
  dimension "d131" = 13
  dimension "d133" = 14
  dimension "d134" = 14
  dimension "d135" = 21
  dimension "d139" = 14
  dimension "d140" = 5
  dimension "d141" = 14
  dimension "d142" = 5
  dimension "d143" = 14
  dimension "d144" = 14
  dimension "d145" = 5
  dimension "d146" = 14
  dimension "d147" = 5
  dimension "d148" = 5
  dimension "d149" = 14
  dimension "d150" = 5
  dimension "d151" = 14
  dimension "d152" = 5
  dimension "d153" = 14
  dimension "d154" = 5
  dimension "d155" = 14
  dimension "d159" = 14
  dimension "d160" = 5
  dimension "d161" = 14
  dimension "d162" = 5
  dimension "d163" = 14
  dimension "d164" = 14
  dimension "d165" = 5
  constraints: 1012 end point, 619 perpendicular, 214 horizontal, 161 point on line, 158 parallel, 27 vertical, 19 collinear, 267 other
  measures "d82" distance of L1.start L19.start
  measures "d83" distance of L1.start L1.end
  measures "d84" distance of L1.end L2.start
  measures "d85" distance of L2.start L2.end
  measures "d86" distance of L2.end L3.start
  measures "d87" distance of L3.start L3.end
  measures "d88" distance of L3.end L4.start
  measures "d89" distance of L4.start L4.end
  measures "d90" distance of L4.end L5.start
  measures "d91" distance of L5.start L5.end
  measures "d92" distance of L5.end L6.start
  measures "d93" distance of L6.start L6.end
  measures "d94" distance of L6.end L7.start
  measures "d95" distance of L7.start L8.start
  measures "d97" distance of L8.end L9.start
  measures "d105" distance of L70.end L35.start
  measures "d106" distance of L35.start L86.end
  measures "d107" distance of L86.end L36.start
  measures "d108" distance of L36.start L36.end
  measures "d109" distance of L36.end L37.start
  measures "d110" distance of L37.start L37.end
  measures "d111" distance of L37.end L38.start
  measures "d112" distance of L38.start L63.end
  measures "d114" distance of L39.start L39.end
  measures "d115" distance of L39.end L40.start
  measures "d116" distance of L40.start L40.end
  measures "d117" distance of L40.end L41.start
  measures "d119" distance of L41.end L42.start
  measures "d120" distance of L42.start L42.end
  measures "d121" distance of L42.end L43.start
  measures "d122" distance of L43.start L43.end
  measures "d123" distance of L43.end L45.start
  measures "d125" distance of L45.start L45.end
  measures "d126" distance of L45.end L48.start
  measures "d127" distance of L48.start L48.end
  measures "d130" distance of L71.end L72.end
  measures "d131" distance of L75.end L77.end
  measures "d133" distance of L31.end L175.start
  measures "d134" distance of L213.end L217.end
  measures "d135" distance of L227.start L227.end
  measures "d139" distance of L233.start L233.end
  measures "d140" distance of L233.end L234.start
  measures "d141" distance of L234.start L234.end
  measures "d142" distance of L234.end L235.start
  measures "d143" distance of L235.start L275.end
  measures "d144" distance of L236.start L236.end
  measures "d145" distance of L236.end L257.start
  measures "d146" distance of L257.start L256.end
  measures "d147" distance of L256.end L238.start
  measures "d148" distance of L254.end L253.start
  measures "d149" distance of L253.start L239.end
  measures "d150" distance of L239.end L240.start
  measures "d151" distance of L240.start L240.end
  measures "d152" distance of L240.end L243.end
  measures "d153" distance of L243.end L309.start
  measures "d154" distance of L309.start L247.start
  measures "d155" distance of L247.start L304.start
  measures "d159" distance of L325.start L325.end
  measures "d160" distance of L325.end L326.start
  measures "d161" distance of L326.start L326.end
  measures "d162" distance of L326.end L327.start
  measures "d163" distance of L327.start L367.end
  measures "d164" distance of L328.start L328.end
  measures "d165" distance of L328.end L349.start
sketch "Sketch15" plane through (0, 18, 0) normal (0, 1, 0) x (1, 0, 0)
  line L0 (-84.1375, -138.1125) -> (-98.425, -138.1125)
  line L1 (-98.425, -138.1125) -> (-98.425, -112.7125)
  line L2 (-98.425, -112.7125) -> (-84.1375, -112.7125)
  line L3 (-84.1375, -112.7125) -> (-84.1375, -138.1125)
  point P0 (0, 0)
  constraints: 8 end point, 2 parallel, 1 horizontal, 1 perpendicular
extrude "Extrusion13" add sketch "Sketch14" along normal blind 2 contours L19 L152 L20 L1 | L21 L156 L22 L2 | L23 L208 L160 L24 L3 | L25 L164 L26 L4 | L27 L211 L168 L28 L5 | L29 L212 L172 L30 L6 | L31 L175 L216 L8 L7 | L222 L214 L10 L217 L218 L9 | L218 L220 L219 | L136 L13 L134 L11 | L14 L140 L15 L138 | L16 L144 L17 L142 | L146 L145 L148 L18 | L48 L49 L128 L50 L32 | L34 L82 L70 L84 L33 | L35 L86 L87 L88 L69 | L36 L67 L92 L68 | L37 L65 L96 L66 | L38 L98 L63 L100 L64 | L39 L61 L104 L62 | L40 L59 L108 L194 L60 | L41 L57 L112 L58 | L42 L55 L116 L56 | L43 L53 L120 L54 | L45 L51 L124 L52 | L71 L72 L73 L74 | L230 L229 L228 L227 | L245 L246 L305 L247 L232 | L235 L275 L260 L277 L261 | L236 L258 L281 L259 | L237 L256 L285 L318 L257 | L238 L254 L289 L255 | L239 L252 L293 L253 | L240 L250 L297 L251 | L242 L248 L301 L249
sketch "Sketch16" plane through (0, 13, 0) normal (0, 1, 0) x (1, 0, 0)
  point P0 (0, 0)
sketch "Sketch17" plane through (0, 18, 0) normal (0, 1, 0) x (1, 0, 0)
  line L0 (-22.225, -134.2875) -> (-22.225, 132.5813) projected
  line L1 (-22.225, -0.8531) -> (-32.225, -0.8531)
  line L2 (-32.225, -0.8531) -> (-32.225, 0)
  line L3 (-32.225, 0) -> (-32.225, 44)
  line L4 (-32.225, 44) -> (-32.225, -44)
  line L5 (-32.225, -44) -> (-47.225, -44)
  line L6 (-47.225, -44) -> (-47.225, 44)
  line L7 (-47.225, 44) -> (-32.225, 44)
  line L8 (-32.225, 44) -> (-32.225, 49)
  line L9 (-32.225, 49) -> (-32.225, 63)
  line L10 (-32.225, 63) -> (-32.225, 68)
  line L11 (-32.225, 68) -> (-32.225, 82)
  line L12 (-32.225, 82) -> (-47.225, 82)
  line L13 (-47.225, 82) -> (-47.225, 68)
  line L14 (-47.225, 68) -> (-32.225, 68)
  line L15 (-47.225, 68) -> (-47.225, 63)
  line L16 (-47.225, 63) -> (-32.225, 63)
  line L17 (-47.225, 63) -> (-47.225, 49)
  line L18 (-47.225, 49) -> (-47.225, 44)
  line L19 (-47.225, 49) -> (-32.225, 49)
  point P0 (0, 0)
  dimension "d198" = 10
  dimension "d199" = 44
  dimension "d200" = 88
  dimension "d201" = 15
  dimension "d202" = 5
  dimension "d203" = 14
  dimension "d204" = 5
  dimension "d205" = 14
  constraints: 38 end point, 9 perpendicular, 7 point on line, 1 collinear, 1 horizontal, 1 midpoint, 1 vertical
  measures "d198" distance of L1.start L1.end
  measures "d199" distance of L2.end L3.end
  measures "d200" distance of L3.end L4.end
  measures "d201" distance of L4.end L5.end
  measures "d202" distance of L3.end L8.end
  measures "d203" distance of L8.end L9.end
  measures "d204" distance of L9.end L10.end
  measures "d205" distance of L10.end L11.end
extrude "Extrusion14" add sketch "Sketch17" along normal blind 2 contours L4 L5 L6 L7 L3 L2 | L19 L17 L16 L9 | L14 L13 L12 L11
sketch "Sketch18" plane through (0, 13, 0) normal (0, 1, 0) x (1, 0, 0)
  line L0 (-120.65, -128.5875) -> (-120.65, -113.5875)
  line L1 (-120.65, -109.5375) -> (-120.65, -125.4125) projected
  line L2 (-120.65, -113.5875) -> (-136.525, -113.5875)
  line L3 (-136.525, -113.5875) -> (-136.525, -128.5875)
  line L4 (-136.525, -125.4125) -> (-136.525, -109.5375) projected
  line L5 (-136.525, -128.5875) -> (-120.65, -128.5875)
  point P0 (0, 0)
  dimension "d208" = 15
  constraints: 8 end point, 2 perpendicular, 1 collinear, 1 point on line
  measures "d208" distance of L0.start L0.end
sketch "Sketch19" plane through (0, 18, 0) normal (0, 1, 0) x (1, 0, 0)
  point P0 (0, 0)
sketch "Sketch20" plane through (0, 18, 0) normal (0, 1, 0) x (1, 0, 0)
  point P0 (0, 0)